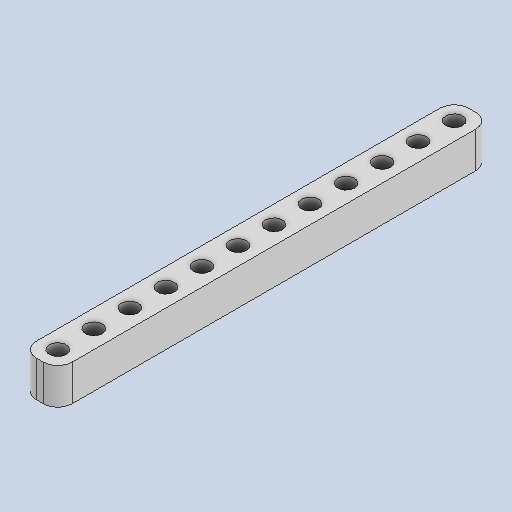
# Autodesk Inventor part: soporte de direccion
Saved by Autodesk Inventor 2024 (Build 280153000, 153)
## iProperties
Created: 2024-03-25
Part Number: soporte de direccion
Material: Generic
Document SubType Name: Modeling
Designer: JDAM
Density: 1 g/cm^3
Appearance: Default
Author: JDAM
Autodesk Inventor part; units mm, degrees
ref_plane "YZ Plane" through (0, 0, 0) normal (1, 0, 0) x (0, 1, 0)
ref_plane "XZ Plane" through (0, 0, 0) normal (0, 1, 0) x (-1, 0, 0)
ref_plane "XY Plane" through (0, 0, 0) normal (0, 0, 1) x (1, 0, 0)
sketch "Sketch1" plane through (0, 0, 0) normal (0, 1, 0) x (-1, 0, 0)
  line L0 (5, 60) -> (-5, 60)
  line L1 (-5, 60) -> (-5, -60)
  line L2 (-5, -60) -> (5, -60)
  line L3 (5, -60) -> (5, 60)
  line L4 (5, 60) -> (-5, -60) construction
  line L5 (-5, 60) -> (5, -60) construction
  point P0 (0, 0)
  dimension "d0" = 10
  dimension "d1" = 120
  constraints: 12 end point, 2 midpoint, 2 parallel, 1 horizontal, 1 perpendicular
  measures "d0" distance of L2.end L1.end
  measures "d1" distance of L1.end L0.end
extrude "Extrusion1" add sketch "Sketch1" along normal blind 10
fillet "Fillet1" radius 4 4 edges at (5, 5, 60) (-5, 5, 60) (-5, 5, -60) (5, 5, -60)
sketch "Sketch2" plane through (0, 10, 0) normal (0, 1, 0) x (1, 0, 0)
  line L0 (1, 60) -> (-1, 60) projected
  line L1 (0, 60) -> (0, -50)
  line L2 (-1, 60) -> (-1, 55)
  arc A0 (-1, 60) -> (-5, 56) centre (-1, 56) ccw projected
  line L3 (-1, 55) -> (0, 55)
  point P0 (0, 0)
  dimension "d5" = 110
  dimension "d6" = 5
  constraints: 6 end point, 2 vertical, 1 midpoint, 1 perpendicular, 1 point on line
  measures "d5" distance of L1.start L1.end
  measures "d6" distance of L0.end L2.end
hole "Hole1" at (0, 10, -55) direction (0, -1, 0) diameter 4.7 depth 12
pattern_linear "Rectangular Pattern1" count 12 spacing 10 along (0, 0, 1) of "Hole1"
body "Solid1"
